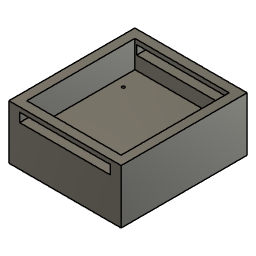
speaker+structure (Autodesk Fusion 360 design; units mm, degrees)
Autodesk Fusion 360 part; units mm, degrees
sketch "Sketch1" plane through (0, 0, 0) normal (0, 1, 0) x (1, 0, 0)
  line L0 (0, 0) -> (150, 0)
  line L1 (150, 0) -> (150, 150)
  line L2 (150, 150) -> (0, 150)
  line L3 (0, 150) -> (0, 0)
  line L4 (0, 0) -> (134.62, 0)
  line L5 (134.62, 0) -> (134.62, 31.75)
  circle A0 centre (134.62, 31.75) radius 1.6
  line L6 (134.62, 0) -> (134.62, 106.68)
  circle A1 centre (134.62, 106.68) radius 1.6
  line L7 (0, 0) -> (50.8, 0)
  line L8 (50.8, 0) -> (50.8, 106.68)
  line L9 (50.8, 0) -> (50.8, 31.75)
  circle A2 centre (50.8, 106.68) radius 1.6
  circle A3 centre (50.8, 31.75) radius 1.6
  dimension "d1" = 150
  dimension "d2" = 150
  dimension "d3" = 134.62
  dimension "d4" = 31.75
  dimension "d5" = 3.2
  dimension "d6" = 106.68
  dimension "d7" = 3.2
  dimension "d8" = 50.8
  dimension "d9" = 106.68
  dimension "d10" = 31.75
  dimension "d11" = 3.2
  dimension "d12" = 3.2
  constraint horizontal L0
  constraint vertical L1
  constraint horizontal L2
  constraint vertical L3
  constraint coincident L0.start L3.end
  constraint perpendicular L3 L4
  constraint perpendicular L4 L5
  constraint coincident L5.end A0.centre
  constraint perpendicular L4 L6
  constraint coincident L6.end A1.centre
  constraint perpendicular L3 L7
  constraint perpendicular L4 L8
  constraint perpendicular L4 L9
  constraint coincident L8.end A2.centre
  constraint coincident L9.end A3.centre
  measures "d1" distance of L0.start L0.end
  measures "d2" distance of L0.start L2.end
  measures "d3" distance of L0.start L4.end
  measures "d4" distance of L4.end L5.end
  measures "d5" diameter of A0
  measures "d6" distance of L4.end L6.end
  measures "d7" diameter of A1
  measures "d8" distance of L0.start L7.end
  measures "d9" distance of L7.end L8.end
  measures "d10" distance of L7.end L9.end
  measures "d11" diameter of A2
  measures "d12" diameter of A3
extrude "Extrude1" add sketch "Sketch1" along normal blind 10
extrude "Extrude2" add 1 faces at (106.3029, 10, -57.1038) along direction (0, 1, 0) blind 20
extrude "Extrude3" cut 1 faces at (0, 10, -100) along direction (1, 0, 0) blind 35.42
extrude "Extrude4" cut 1 faces at (111.8067, 10, -150) along direction (0, 0, 1) blind 10.17
extrude "Extrude5" add 1 faces at (35.42, 10, -93.22) along direction (-1, 0, 0) blind 5
extrude "Extrude6" add 1 faces at (150, 10, -46.61) along direction (1, 0, 0) blind 5
sketch "Sketch2" plane through (0, 30, 0) normal (0, 1, 0) x (-1, 0, 0)
  circle A0 centre (-50.8, -106.68) radius 1.6
  circle A1 centre (-134.62, -31.75) radius 1.6
  circle A2 centre (-50.8, -31.75) radius 1.6
  circle A3 centre (-134.62, -106.68) radius 1.6
  line L0 (-155, -139.83) -> (-30.42, -139.83)
  line L1 (-30.42, -139.83) -> (-30.42, 0)
  line L2 (-30.42, 0) -> (-155, 0)
  line L3 (-155, 0) -> (-155, -139.83)
  line L4 (-30.42, -139.83) -> (-30.42, -129.83)
  line L5 (-155, 0) -> (-145, 0)
  line L6 (-40.42, -129.83) -> (-145, -129.83)
  line L7 (-145, -129.83) -> (-145, -10)
  line L8 (-145, -10) -> (-40.42, -10)
  line L9 (-40.42, -10) -> (-40.42, -129.83)
  dimension "d26" = 10
  dimension "d27" = 10
  constraint coincident L0.end L1.start
  constraint perpendicular L0 L4
  constraint coincident L2.end L3.start
  constraint perpendicular L3 L5
  constraint horizontal L6
  constraint vertical L7
  constraint horizontal L8
  constraint vertical L9
  measures "d26" distance of L4.end L6.start
  measures "d27" distance of L2.end L5.end
extrude "Extrude7" add sketch "Sketch2" along normal blind 30 contours L0 L1 L2 L3 L4 L5
sketch "Sketch3" plane through (0, 0, -139.83) normal (0, 0, -1) x (-1, 0, 0)
  line L0 (-155, 60) -> (-155, 0)
  line L1 (-155, 0) -> (-30.42, 0)
  line L2 (-30.42, 0) -> (-30.42, 60)
  line L3 (-30.42, 60) -> (-155, 60)
  line L4 (-155, 60) -> (-155, 55)
  line L5 (-155, 55) -> (-143, 55)
  line L6 (-30.42, 60) -> (-30.42, 55)
  line L7 (-30.42, 55) -> (-42.42, 55)
  line L8 (-42.42, 55) -> (-42.42, 45)
  line L9 (-143, 55) -> (-42.42, 55)
  line L10 (-42.42, 55) -> (-42.42, 45)
  line L11 (-42.42, 45) -> (-143, 45)
  line L12 (-143, 45) -> (-143, 55)
  dimension "d30" = 12
  dimension "d31" = 12
  constraint coincident L0.start L3.end
  constraint coincident L0 L4.end
  constraint perpendicular L3 L4
  constraint perpendicular L4 L5
  constraint coincident L2.end L3.start
  constraint coincident L2 L6.end
  constraint perpendicular L3 L6
  constraint perpendicular L2 L7
  constraint perpendicular L7 L8
  constraint horizontal L9
  constraint vertical L10
  constraint horizontal L11
  constraint vertical L12
  measures "d30" distance of L4.end L5.end
  measures "d31" distance of L6.end L7.end
extrude "Extrude8" cut sketch "Sketch3" against normal blind 200 contours L8 L9 L10 L11 L12
